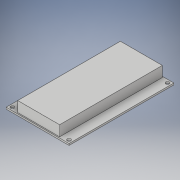
# Autodesk Inventor part: LCD Screen
Saved by Autodesk Inventor 2019 (Build 230136000, 136)
## iProperties
Created: 2019-03-10
Part Number: LCD Screen
Material: Generic
Document SubType Name: Modeling
Designer: savo
Density: 1 g/cm^3
Appearance: Default
Author: savo
Autodesk Inventor part; units mm, degrees
ref_plane "YZ Plane" through (0, 0, 0) normal (1, 0, 0) x (0, 1, 0)
ref_plane "XZ Plane" through (0, 0, 0) normal (0, 1, 0) x (-1, 0, 0)
ref_plane "XY Plane" through (0, 0, 0) normal (0, 0, 1) x (1, 0, 0)
sketch "Sketch1" plane through (0, 0, 0) normal (0, 1, 0) x (-1, 0, 0)
  line L0 (0, 0) -> (60, 0)
  line L1 (60, 0) -> (60, -100)
  line L2 (60, -100) -> (0, -100)
  line L3 (0, -100) -> (0, 0)
  dimension "d0" = 60
  dimension "d1" = 100
  constraints: 8 end point, 2 parallel, 1 horizontal, 1 perpendicular
  measures "d0" distance of L1.end L2.end
  measures "d1" distance of L0.end L1.end
extrude "Extrusion1" add sketch "Sketch1" along normal blind 1.6
sketch "Sketch2" plane through (0, 1.6, 0) normal (0, 1, 0) x (1, 0, 0)
  line L0 (-60, 0) -> (0, 0) projected
  line L1 (0, 0) -> (0, 100) projected
  point P0 (-3, 3)
  point P1 (-57, 3)
  point P2 (-3, 97)
  point P3 (-57, 97)
  dimension "d4" = 3
  dimension "d5" = 3
  dimension "d8" = 54
  dimension "d11" = 94
  constraints: 1 horizontal, 1 vertical, 3 other
  measures "d4" distance from line of L0 point (-3, 3)
  measures "d5" distance from line of L1 point (-3, 3)
  measures "d8" distance of point (-3, 3) point (-57, 3)
  measures "d11" distance of point (-3, 3) point (-3, 97)
hole "Hole1" at (-3, 1.6, -3) at (-57, 1.6, -3) at (-3, 1.6, -97) at (-57, 1.6, -97) direction (0, -1, 0) diameter 3.4 end through all clearance for "Flat Head Machine Screw" size "M3" standard "Ansi Metric M Profile"
sketch "Sketch3" plane through (0, 1.6, 0) normal (0, 1, 0) x (1, 0, 0)
  line L0 (0, 0) -> (-60, 0) construction
  line L1 (-30, 0) -> (-30, 100) construction
  line L2 (-60, 100) -> (0, 100) construction
  line L3 (-50, 1) -> (-10, 1)
  line L4 (-10, 1) -> (-10, 99)
  line L5 (-10, 99) -> (-50, 99)
  line L6 (-50, 99) -> (-50, 1)
  line L7 (-50, 1) -> (-10, 99) construction
  point P0 (-30, 50)
  dimension "d21" = 40
  dimension "d22" = 98
  constraints: 12 end point, 4 midpoint, 2 parallel, 1 horizontal, 1 perpendicular
  measures "d21" distance of L5.end L4.end
  measures "d22" distance of L4.end L3.end
extrude "Extrusion2" add sketch "Sketch3" along normal blind 10
body "Solid1"
